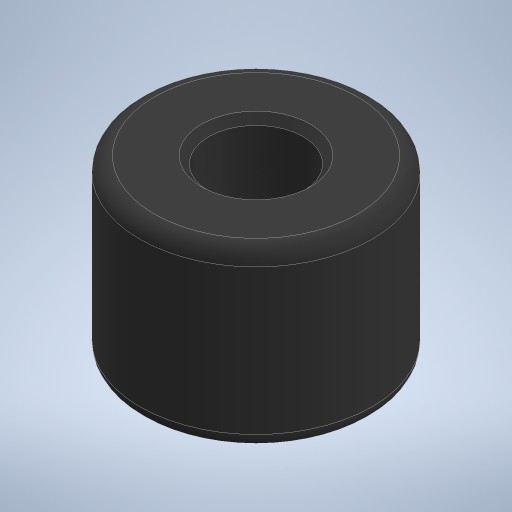
# Autodesk Inventor part: REVO-heater
Saved by Autodesk Inventor 2023.1 (Build 271208000, 208)
## iProperties
Created: 2022-11-20
Part Number: REVO-heater
Material: Rubber
Document SubType Name: Modeling
Designer: Frank
Density: 0.93 g/cm^3
Appearance: Rubber - Black
Mass: 1.84903 g
Surface Area: 11.2864 cm^2
Volume: 1.98821 cm^3
Author: Frank
Autodesk Inventor part; units mm, degrees
ref_plane "YZ Plane" through (0, 0, 0) normal (1, 0, 0) x (0, 1, 0)
ref_plane "XZ Plane" through (0, 0, 0) normal (0, 1, 0) x (-1, 0, 0)
ref_plane "XY Plane" through (0, 0, 0) normal (0, 0, 1) x (1, 0, 0)
sketch "Sketch1" plane through (0, 0, 0) normal (0, 0, 1) x (1, 0, 0)
  line L0 (0, 6) -> (-8, 6)
  line L1 (-8, 6) -> (-8, -6)
  line L2 (-8, -6) -> (0, -6)
  line L3 (0, -6) -> (0, 6)
  line L4 (-3.25, 6) -> (-3.25, -6)
  point P0 (0, 0)
  point P1 (0, 0)
  dimension "d0" = 12
  dimension "d1" = 6.5
  dimension "d2" = 16
  constraints: 10 end point, 2 parallel, 2 perpendicular, 2 point on line, 1 coincident, 1 horizontal, 1 midpoint
  measures "d0" distance of L2.end L0.start
  measures "d1" diameter of L4 L3
  measures "d2" diameter of L1 L3
revolve "Revolution1" add sketch "Sketch1" angle 360 about axis through (0, -6, 0) along (0, 1, 0) contours L4 L2 L1 L0
fillet "Fillet1" radius 1 2 edges at (8, 6, 0) (8, -6, 0)
chamfer "Chamfer1" distance 0.5 angle 45 2 edges at (3.25, 6, 0) (3.25, -6, 0)
body "Solid1"
